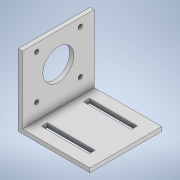
# Autodesk Inventor part: Metal_AttachmentBracket
Saved by Autodesk Inventor 2022 (Build 260153000, 153)
## iProperties
Created: 2022-02-26
Part Number: Metal_AttachmentBracket
Material: Generic
Document SubType Name: Modeling
Designer: Mlees
Density: 1 g/cm^3
Appearance: Default
Author: Mlees
Autodesk Inventor part; units mm, degrees
ref_plane "YZ Plane" through (0, 0, 0) normal (1, 0, 0) x (0, 1, 0)
ref_plane "XZ Plane" through (0, 0, 0) normal (0, 1, 0) x (-1, 0, 0)
ref_plane "XY Plane" through (0, 0, 0) normal (0, 0, 1) x (1, 0, 0)
sketch "Sketch1" plane through (0, 0, 0) normal (0, 0, 1) x (1, 0, 0)
  line L0 (0, 0) -> (0, 51)
  line L1 (0, 51) -> (3, 51)
  line L2 (3, 51) -> (3, 3)
  line L3 (3, 3) -> (51, 3)
  line L4 (51, 3) -> (51, 0)
  line L5 (51, 0) -> (0, 0)
  dimension "d0" = 51
  dimension "d1" = 3
  dimension "d2" = 48
  dimension "d3" = 48
  constraints: 12 end point, 5 perpendicular, 1 vertical
  measures "d0" distance of L0.start L0.end
  measures "d1" distance of L0.end L1.end
  measures "d2" distance of L1.end L2.end
  measures "d3" distance of L2.end L3.end
extrude "Extrusion1" add sketch "Sketch1" along normal blind 51
sketch "Sketch2" plane through (3, 3, 0) normal (1, 0, 0) x (0, 0, -1)
  line L0 (0, 48) -> (-51, 48) projected
  circle A0 centre (-25.5, 27) radius 11
  circle A1 centre (-41, 42.5) radius 1.5
  circle A2 centre (-10, 42.5) radius 1.5
  circle A3 centre (-10, 11.5) radius 1.5
  circle A4 centre (-41, 11.5) radius 1.5
  point P0 (0, -3)
  dimension "d7" = 22
  dimension "d12" = 3
  dimension "d13" = 3
  constraints: 5 centre point
  measures "d7" diameter of A0
  measures "d12" diameter of A1
  measures "d13" diameter of A2
extrude "Extrusion2" cut sketch "Sketch2" against normal up to surface (3 mm away)
sketch "Sketch3" plane through (3, 3, 0) normal (0, 1, 0) x (1, 0, 0)
  line L0 (48, 0) -> (48, -51) projected
  line L1 (48, -25.5) -> (48, -12.635)
  line L2 (48, -12.635) -> (48, -10.485)
  line L3 (48, -10.485) -> (39, -10.485)
  line L4 (-3, 0) -> (48, 0) projected
  line L5 (39, 0) -> (39, -7.85)
  line L6 (39, 0) -> (46.85, 0) construction
  line L7 (39, -10.485) -> (39, -8.335)
  line L8 (39, -8.335) -> (5, -8.335)
  line L9 (5, -8.335) -> (5, -12.635)
  line L10 (5, -12.635) -> (39, -12.635)
  line L11 (39, -12.635) -> (39, -10.485)
  line L12 (48, -25.5) -> (-0.1529, -25.5)
  line L13 (39, -40.515) -> (39, -42.665)
  line L14 (39, -42.665) -> (5, -42.665)
  line L15 (5, -42.665) -> (5, -38.365)
  line L16 (5, -38.365) -> (39, -38.365)
  line L17 (39, -38.365) -> (39, -40.515)
  point P0 (39, -43.15)
  dimension "d16" = 12.865
  dimension "d17" = 2.15
  dimension "d18" = 9
  dimension "d20" = 7.85
  dimension "d21" = 270
  dimension "d22" = 2.15
  dimension "d23" = 4.3
  constraints: 32 end point, 6 perpendicular, 6 symmetric about line, 5 point on line, 3 horizontal, 1 midpoint, 1 vertical
  measures "d16" distance of L1.start L1.end
  measures "d17" distance of L1.end L2.end
  measures "d18" distance of L2.end L3.end
  measures "d20" distance of L5.start L5.end
  measures "d22" distance of L3.end L7.end
  measures "d23" distance of L8.end L9.end
extrude "Extrusion3" cut sketch "Sketch3" against normal through all
body "Solid1"
